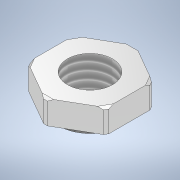
# Autodesk Inventor part: S4-07-3W
Saved by Autodesk Inventor 2020 (Build 240168000, 168)
## iProperties
Created: 2021-09-02
Part Number: S4-07-3W
Material: ステンレス鋼 AISI 304
Document SubType Name: Modeling
Designer: naoki
Density: 8 g/cm^3
Appearance: クロム - サテン
Mass: 0.368542 g
Surface Area: 1.13119 cm^2
Volume: 0.0460677 cm^3
Description: 既製品
Author: Naoki Iwasawa
Comments: https://jp.misumi-ec.com/vona2/detail/221000555662/?PNSearch=S4-07-3W&HissuCode=S4-07-3W
Autodesk Inventor part; units mm, degrees
ref_plane "YZ Plane" through (0, 0, 0) normal (1, 0, 0) x (0, 1, 0)
ref_plane "XZ Plane" through (0, 0, 0) normal (0, 1, 0) x (-1, 0, 0)
ref_plane "XY Plane" through (0, 0, 0) normal (0, 0, 1) x (1, 0, 0)
sketch "スケッチ2" plane through (0, 0, 0) normal (0, 1, 0) x (-1, 0, 0)
  circle A0 centre (0, 0) radius 2
  circle A1 centre (0, 0) radius 2.75
  circle A2 centre (0, 0) radius 3.5
  line L0 (3.2709, 0) -> (-4.3069, 0) construction
  line L1 (-3.5, -2.0207) -> (0, -4.0415)
  line L2 (-3.5, 0) -> (-3.5, -2.0207)
  line L3 (0, 3.4516) -> (0, -4.8702) construction
  line L4 (-3.5, 2.0207) -> (0, 4.0415)
  line L5 (-3.5, 0) -> (-3.5, 2.0207)
  line L6 (3.5, -2.0207) -> (0, -4.0415)
  line L7 (3.5, 0) -> (3.5, -2.0207)
  line L8 (3.5, 2.0207) -> (0, 4.0415)
  line L9 (3.5, 0) -> (3.5, 2.0207)
  dimension "d8" = 7
  dimension "d6" = 4
  dimension "d7" = 5.5
  dimension "d25" = 120
  constraints: 20 end point, 5 symmetric about line, 3 coincident, 3 vertical, 2 centre point, 2 point on line, 1 horizontal, 1 horizontal alignment, 1 perpendicular, 4 other
  measures "d6" diameter of A0
  measures "d7" diameter of A1
  measures "d25" angle of L2 L1
extrude "押し出し1" add sketch "スケッチ2" against normal blind 0.7 contours A1
extrude "押し出し2" add sketch "スケッチ2" along normal blind 2.1 contours A1 | A2 | L7 L6 A2 | A2 L8 L9 | A2 L4 L8 | L6 L1 A2 | A2 L5 L4 | L1 L2 A2
chamfer "面取り1" distance 0.2 angle 45 6 edges at (3.5, 1.05, -2.0207) (0, 1.05, -4.0415) (-3.5, 1.05, -2.0207) (-3.5, 1.05, 2.0207) (0, 1.05, 4.0415) (3.5, 1.05, 2.0207)
chamfer "面取り2" distance 0.2 angle 45 6 edges at (3.4134, 2.1, -1.9707) (0, 2.1, -3.9415) (-3.4134, 2.1, -1.9707) (-3.4134, 2.1, 1.9707) (0, 2.1, 3.9415) (3.4134, 2.1, 1.9707)
thread "ねじ1" size "M4x0.7" class "6H" standard "ANSI Metric M Profile" full length
